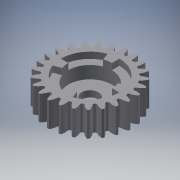
# Autodesk Inventor part: gear 3 clutch herring
Saved by Autodesk Inventor 2017 (Build 210142000, 142)
## iProperties
Created: 2018-04-17
Part Number: gear 3 clutch herring
Material: Generic
Document SubType Name: Modeling
Designer: RKL
Density: 1 g/cm^3
Appearance: Default
Author: RKL
Autodesk Inventor part; units mm, degrees
ref_plane "YZ Plane" through (0, 0, 0) normal (1, 0, 0) x (0, 1, 0)
ref_plane "XZ Plane" through (0, 0, 0) normal (0, 1, 0) x (-1, 0, 0)
ref_plane "XY Plane" through (0, 0, 0) normal (0, 0, 1) x (1, 0, 0)
sketch "Sketch1" plane through (0, 0, 0) normal (0, 0, 1) x (1, 0, 0)
  spline S0 degree 3 poles (-3.4503, 33.5732) (-3.2826, 33.3305) (-2.9471, 32.8453) (-2.5006, 32.0808) (-2.102, 31.2901) (-1.7718, 30.4694) (-1.5576, 29.7602) (-1.4857, 29.1741) (-1.3672, 28.7464) (-1.2008, 28.4129) (-1.0111, 28.1856) (-0.8419, 28.0424) (-0.6545, 27.9224) (-0.3696, 27.8358) (0, 27.8305) (0.3696, 27.8358) (0.6545, 27.9224) (0.8419, 28.0424) (1.0111, 28.1856) (1.2008, 28.4129) (1.3672, 28.7464) (1.4857, 29.1741) (1.5576, 29.7602) (1.7718, 30.4694) (2.102, 31.2901) (2.5006, 32.0808) (2.9471, 32.8453) (3.2826, 33.3305) (3.4503, 33.5732) knots 0 0 0 0 0.088459 0.176919 0.265374 0.353819 0.442221 0.486455 0.530676 0.574845 0.596976 0.619041 0.641139 0.663246 0.707314 0.751382 0.773488 0.795586 0.817652 0.839782 0.883952 0.928172 0.972406 1.060809 1.149253 1.237709 1.326168 1.414628 1.414628 1.414628 1.414628
  circle A0 centre (0, 0) radius 27.8326 construction
  circle A1 centre (0, 0) radius 29.3654 construction
  circle A2 centre (0, 0) radius 31.25 construction
  circle A3 centre (0, 0) radius 33.75
  point P0 (-2.9566, 32.8392)
  point P1 (-2.5086, 32.0764)
  point P2 (-2.1134, 31.285)
  point P3 (-1.7839, 30.4642)
  point P4 (-1.5479, 29.6123)
  point P5 (-1.4749, 29.176)
  point P6 (-1.3536, 28.7508)
  point P7 (-1.1487, 28.3595)
  point P8 (-1.0064, 28.19)
  point P9 (-0.8389, 28.0463)
  point P10 (-0.6501, 27.9316)
  point P11 (-0.4395, 27.8642)
  point P12 (0, 27.8326)
  point P13 (0.4395, 27.8642)
  point P14 (0.6501, 27.9316)
  point P15 (0.8389, 28.0463)
  point P16 (1.0064, 28.19)
  point P17 (1.1487, 28.3595)
  point P18 (1.3536, 28.7508)
  point P19 (1.4749, 29.176)
  point P20 (1.5479, 29.6123)
  point P21 (1.7839, 30.4642)
  point P22 (2.1134, 31.285)
  point P23 (2.5086, 32.0764)
  point P24 (2.9566, 32.8392)
  constraints: 4 centre point, 2 point on circle, 59 other
extrude "Extrusion1" add sketch "Sketch1" against normal blind 20
extrude "Extrusion2" cut sketch "Sketch1" against normal through all contours A3 S0 picked at (-0.5327, 31.9242)
pattern_circular "Circular Pattern1" count 25 over 360 about axis through (0, 0, 0) along (0, 0, -1) of "Extrusion2"
sketch "Sketch2" plane through (0, 0, 0) normal (0, 0, 1) x (1, 0, 0)
  circle A0 centre (0, 0) radius 6.75
  dimension "d7" = 13.5
  constraints: 1 centre point, 1 coincident
  measures "d7" diameter of A0
extrude "Extrusion3" cut sketch "Sketch2" against normal through all
sketch "Sketch3" plane through (0, 0, 0) normal (0, 0, 1) x (1, 0, 0)
  circle A0 centre (0, 0) radius 17.5
  dimension "d10" = 35
  constraints: 1 centre point, 1 coincident
  measures "d10" diameter of A0
extrude "Extrusion4" cut sketch "Sketch3" against normal blind 15
sketch "Sketch4" plane through (0, 0, 0) normal (0, 0, 1) x (1, 0, 0)
  circle A0 centre (0, 0) radius 17.5 construction
  line L0 (0, 0) -> (0, 17.5) construction
  line L1 (0, 17.5) -> (0, 23.5)
  arc A1 (22.0828, 8.0375) -> (0, 23.5) centre (0, 0) ccw
  arc A2 (16.4446, 5.9854) -> (0, 17.5) centre (0, 0) ccw
  line L2 (22.0828, 8.0375) -> (16.4446, 5.9854)
  dimension "d13" = 6
  dimension "d14" = 70
  constraints: 6 end point, 4 point on circle, 2 centre point, 2 coincident, 1 line through centre, 1 point on line, 1 vertical, 1 vertical alignment, 1 other
  measures "d13" distance of L0.end L1.end
  measures "d14" angle of L2 L1
extrude "Extrusion5" cut sketch "Sketch4" against normal blind 5
pattern_circular "Circular Pattern2" count 4 over 360 about axis through (0, 0, 0) along (0, 0, -1) of "Extrusion5"
equation "\"d0\" = FaceWidth"
equation "\"Module\" = 2.5"
equation "\"PressureAngle\" = 20deg"
equation "\"UnitProfileClearance\" = 0.25"
equation "\"UnitRoundRadius\" = 0.35"
equation "\"HeadDiameter\" = 67.5"
equation "\"RootDiameter\" = 55.66524"
equation "\"BaseDiameter\" = 58.73079"
equation "\"PitchDiameter\" = 62.5"
equation "\"FaceWidth\" = 20"
equation "\"HelixAngle\" = 0"
equation "\"UnitCorrection\" = 0"
equation "\"UnitAddendumModification\" = 0"
equation "\"CircularPitch\" = 7.853982"
equation "\"UnitBacklashShift\" = -0.116952"
equation "\"TotalToolShift\" = -0.29238"
equation "\"IsInternal\" = 0"
body "Solid1"
